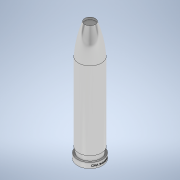
# Autodesk Inventor part: Bala do revólver
Saved by Autodesk Inventor 2021 (Build 250183000, 183)
## iProperties
Created: 2020-11-05
Part Number: Bala do revólver
Material: Liga de Nickel-Copper 400
Document SubType Name: Modeling
Designer: Bruno
Density: 8.83 g/cm^3
Appearance: Cromado - Polido
Author: Bruno
Autodesk Inventor part; units mm, degrees
note: some values were not read from the file. Chosen so that the rebuilt part matches the saved one: direction of "Relevo1".
ref_plane "XY Plane" through (0, 0, 0) normal (0, 0, 1) x (1, 0, 0)
sketch "Esboço1" plane through (0, 0, 0) normal (0, 1, 0) x (-1, 0, 0)
  circle A0 centre (0, 0) radius 3.5
  dimension "d0" = 7
  constraints: 1 centre point, 1 coincident
  measures "d0" diameter of A0
extrude "Extrusão1" add sketch "Esboço1" along normal blind 1.5
sketch "Esboço2" plane through (0, 1.5, 0) normal (0, 1, 0) x (1, 0, 0)
  circle A0 centre (0, 0) radius 3
  dimension "d3" = 6
  constraints: 1 centre point, 1 coincident
  measures "d3" diameter of A0
extrude "Extrusão2" add sketch "Esboço2" along normal blind 1.5
sketch "Esboço3" plane through (0, 3, 0) normal (0, 1, 0) x (1, 0, 0)
  circle A0 centre (0, 0) radius 3.25
  dimension "d6" = 6.5
  constraints: 1 centre point, 1 coincident
  measures "d6" diameter of A0
extrude "Extrusão3" add sketch "Esboço3" along normal blind 22
sketch "Esboço4" plane through (0, 0, 0) normal (0, 0, 1) x (1, 0, 0)
  line L0 (0, 25) -> (0, 36.9625)
  line L1 (0, -7.4277) -> (0, 44.566) projected
  line L2 (3.25, 25) -> (-3.25, 25) projected
  line L3 (0, 25) -> (3.25, 25)
  arc A0 (3.25, 25) -> (0, 36.9625) centre (-25.6934, 23.5594) ccw
  point P0 (0, 0)
  constraints: 4 end point, 2 point on circle, 1 centre point, 1 horizontal, 1 vertical
revolve "Revolução2" add sketch "Esboço4" angle 360 about axis through (0, -10, 0) along (0, 1, 0)
ref_plane "Plano de trabalho1" through (0, 36.963, 0) normal (0, 1, 0) x (-1, 0, 0)
sketch "Esboço5" plane through (0, 36.963, 0) normal (0, 1, 0) x (-1, 0, 0)
  circle A0 centre (0, 0) radius 1.5
  dimension "d12" = 3
  constraints: 1 centre point, 1 coincident
  measures "d12" diameter of A0
extrude "Extrusão4" cut sketch "Esboço5" against normal blind 3.963
sketch "Esboço6" plane through (0, 0, 0) normal (0, -1, 0) x (1, 0, 0)
  circle A0 centre (0, 0) radius 1.25
  dimension "d15" = 2.5
  constraints: 1 centre point, 1 coincident
  measures "d15" diameter of A0
extrude "Extrusão5" cut sketch "Esboço6" against normal blind 0.5
sketch "Esboço7" plane through (0, 0.5, 0) normal (0, -1, 0) x (1, 0, 0)
  circle A0 centre (0, 0) radius 1.25 projected
  circle A1 centre (0, 0) radius 1.2
  dimension "d18" = 2.4
  constraints: 1 centre point, 1 coincident
  measures "d18" diameter of A1
extrude "Extrusão6" add sketch "Esboço7" along normal blind 0.5 contours A1
sketch "Esboço8" plane through (0, 0, 0) normal (0, -1, 0) x (1, 0, 0)
  circle A0 centre (0, 0) radius 0.05
  dimension "d21" = 0.1
  constraints: 1 centre point, 1 coincident
  measures "d21" diameter of A0
extrude "Extrusão7" cut sketch "Esboço8" against normal blind 0.5
ref_plane "Plano de trabalho2" through (3.5, 0, 0) normal (1, 0, 0) x (0, 1, 0)
sketch "Esboço10" plane through (3.5, 0, 0) normal (1, 0, 0) x (0, 1, 0)
  line L0 (0.9718, 2.3396) -> (0.9718, -2.2443) construction
  line L1 (0.9718, -2.2443) -> (0.439, -2.2443) construction
  line L2 (0.439, -2.2443) -> (0.439, 2.3396) construction
  line L3 (0.439, 2.3396) -> (0.9718, 2.3396) construction
  spline S0 degree 2 poles (0.4406, 2.0936) (0.4406, 2.1422) (0.4735, 2.2245) (0.5063, 2.2545) knots 0 0 0 1 2 2 2
  spline S1 degree 2 poles (0.5063, 2.2545) (0.5387, 2.2845) (0.6359, 2.3173) (0.6991, 2.3173) knots 0 0 0 1 2 2 2
  spline S2 degree 2 poles (0.6991, 2.3173) (0.7619, 2.3173) (0.8551, 2.2853) (0.8896, 2.2549) knots 0 0 0 1 2 2 2
  spline S3 degree 2 poles (0.8896, 2.2549) (0.9232, 2.2249) (0.9585, 2.1431) (0.9585, 2.0924) knots 0 0 0 1 2 2 2
  spline S4 degree 2 poles (0.9585, 2.0924) (0.9585, 2.0673) (0.9512, 2.0231) (0.9455, 2.0045) knots 0 0 0 1 2 2 2
  spline S5 degree 2 poles (0.9455, 2.0045) (0.9402, 1.9883) (0.9252, 1.9546) (0.9163, 1.938) knots 0 0 0 1 2 2 2
  line L4 (0.9163, 1.938) -> (0.8361, 1.938)
  line L5 (0.8361, 1.938) -> (0.8361, 1.9433)
  spline S6 degree 2 poles (0.8361, 1.9433) (0.8442, 1.9522) (0.8669, 1.9798) (0.8778, 1.9996) knots 0 0 0 1 2 2 2
  spline S7 degree 2 poles (0.8778, 1.9996) (0.8884, 2.0187) (0.9017, 2.0636) (0.9017, 2.0928) knots 0 0 0 1 2 2 2
  spline S8 degree 2 poles (0.9017, 2.0928) (0.9017, 2.1248) (0.8754, 2.182) (0.8503, 2.2034) knots 0 0 0 1 2 2 2
  spline S9 degree 2 poles (0.8503, 2.2034) (0.8247, 2.2245) (0.7474, 2.248) (0.6991, 2.248) knots 0 0 0 1 2 2 2
  spline S10 degree 2 poles (0.6991, 2.248) (0.6477, 2.248) (0.5735, 2.2233) (0.548, 2.2018) knots 0 0 0 1 2 2 2
  spline S11 degree 2 poles (0.548, 2.2018) (0.5233, 2.1807) (0.4982, 2.1244) (0.4982, 2.0928) knots 0 0 0 1 2 2 2
  spline S12 degree 2 poles (0.4982, 2.0928) (0.4982, 2.064) (0.5124, 2.015) (0.5229, 1.996) knots 0 0 0 1 2 2 2
  spline S13 degree 2 poles (0.5229, 1.996) (0.5334, 1.9777) (0.5553, 1.9506) (0.563, 1.9429) knots 0 0 0 1 2 2 2
  line L6 (0.563, 1.9429) -> (0.563, 1.938)
  line L7 (0.563, 1.938) -> (0.4836, 1.938)
  spline S14 degree 2 poles (0.4836, 1.938) (0.4759, 1.9546) (0.4617, 1.9838) (0.4552, 2.0045) knots 0 0 0 1 2 2 2
  spline S15 degree 2 poles (0.4552, 2.0045) (0.4479, 2.0264) (0.4406, 2.0636) (0.4406, 2.0936) knots 0 0 0 1 2 2 2
  line L8 (0.4495, 1.4473) -> (0.4495, 1.5138)
  line L9 (0.4495, 1.5138) -> (0.8803, 1.5138)
  line L10 (0.8803, 1.5138) -> (0.5873, 1.6443)
  line L11 (0.5873, 1.6443) -> (0.5873, 1.6848)
  line L12 (0.5873, 1.6848) -> (0.8803, 1.814)
  line L13 (0.8803, 1.814) -> (0.4495, 1.814)
  line L14 (0.4495, 1.814) -> (0.4495, 1.876)
  line L15 (0.4495, 1.876) -> (0.9495, 1.876)
  line L16 (0.9495, 1.876) -> (0.9495, 1.7853)
  line L17 (0.9495, 1.7853) -> (0.6712, 1.6605)
  line L18 (0.6712, 1.6605) -> (0.9495, 1.5397)
  line L19 (0.9495, 1.5397) -> (0.9495, 1.4473)
  line L20 (0.9495, 1.4473) -> (0.4495, 1.4473)
  line L21 (0.4495, 1.3999) -> (0.9495, 1.2314)
  line L22 (0.9495, 1.2314) -> (0.9495, 1.1495)
  line L23 (0.9495, 1.1495) -> (0.4495, 0.981)
  line L24 (0.4495, 0.981) -> (0.4495, 1.0511)
  line L25 (0.4495, 1.0511) -> (0.5893, 1.0965)
  line L26 (0.5893, 1.0965) -> (0.5893, 1.2873)
  line L27 (0.5893, 1.2873) -> (0.4495, 1.3327)
  line L28 (0.4495, 1.3327) -> (0.4495, 1.3999)
  line L29 (0.6461, 1.1147) -> (0.8815, 1.1921)
  line L30 (0.8815, 1.1921) -> (0.6461, 1.2691)
  line L31 (0.6461, 1.2691) -> (0.6461, 1.1147)
  line L32 (0.4495, 0.5446) -> (0.4495, 0.7383)
  line L33 (0.4495, 0.7383) -> (0.5006, 0.7383)
  line L34 (0.5006, 0.7383) -> (0.5006, 0.6747)
  line L35 (0.5006, 0.6747) -> (0.8985, 0.6747)
  line L36 (0.8985, 0.6747) -> (0.8985, 0.7383)
  line L37 (0.8985, 0.7383) -> (0.9495, 0.7383)
  line L38 (0.9495, 0.7383) -> (0.9495, 0.5446)
  line L39 (0.9495, 0.5446) -> (0.8985, 0.5446)
  line L40 (0.8985, 0.5446) -> (0.8985, 0.6082)
  line L41 (0.8985, 0.6082) -> (0.5006, 0.6082)
  line L42 (0.5006, 0.6082) -> (0.5006, 0.5446)
  line L43 (0.5006, 0.5446) -> (0.4495, 0.5446)
  line L44 (0.4495, 0.1726) -> (0.4495, 0.2358)
  line L45 (0.4495, 0.2358) -> (0.6635, 0.2358)
  spline S16 degree 2 poles (0.6635, 0.2358) (0.6894, 0.2358) (0.734, 0.2407) (0.7474, 0.248) knots 0 0 0 1 2 2 2
  spline S17 degree 2 poles (0.7474, 0.248) (0.7615, 0.2557) (0.7753, 0.2832) (0.7753, 0.3067) knots 0 0 0 1 2 2 2
  spline S18 degree 2 poles (0.7753, 0.3067) (0.7753, 0.3302) (0.7502, 0.3801) (0.7299, 0.404) knots 0 0 0 1 2 2 2
  line L46 (0.7299, 0.404) -> (0.4495, 0.404)
  line L47 (0.4495, 0.404) -> (0.4495, 0.4672)
  line L48 (0.4495, 0.4672) -> (0.8247, 0.4672)
  line L49 (0.8247, 0.4672) -> (0.8247, 0.404)
  line L50 (0.8247, 0.404) -> (0.783, 0.404)
  spline S19 degree 2 poles (0.783, 0.404) (0.8085, 0.3756) (0.8353, 0.3209) (0.8353, 0.2901) knots 0 0 0 1 2 2 2
  spline S20 degree 2 poles (0.8353, 0.2901) (0.8353, 0.235) (0.7624, 0.1726) (0.6931, 0.1726) knots 0 0 0 1 2 2 2
  line L51 (0.6931, 0.1726) -> (0.4495, 0.1726)
  line L52 (0.4495, -0.2046) -> (0.4495, -0.1414)
  line L53 (0.4495, -0.1414) -> (0.4876, -0.1414)
  spline S21 degree 2 poles (0.4876, -0.1414) (0.4755, -0.1268) (0.4593, -0.1053) (0.4524, -0.0907) knots 0 0 0 1 2 2 2
  spline S22 degree 2 poles (0.4524, -0.0907) (0.4459, -0.0774) (0.439, -0.0486) (0.439, -0.0296) knots 0 0 0 1 2 2 2
  spline S23 degree 2 poles (0.439, -0.0296) (0.439, 0.0012) (0.4645, 0.0531) (0.4893, 0.0713) knots 0 0 0 1 2 2 2
  spline S24 degree 2 poles (0.4893, 0.0713) (0.514, 0.0896) (0.5869, 0.1098) (0.6343, 0.1098) knots 0 0 0 1 2 2 2
  spline S25 degree 2 poles (0.6343, 0.1098) (0.6837, 0.1098) (0.7559, 0.0843) (0.783, 0.062) knots 0 0 0 1 2 2 2
  spline S26 degree 2 poles (0.783, 0.062) (0.8073, 0.0414) (0.8353, -0.0166) (0.8353, -0.0486) knots 0 0 0 1 2 2 2
  spline S27 degree 2 poles (0.8353, -0.0486) (0.8353, -0.0766) (0.8227, -0.1183) (0.8098, -0.1414) knots 0 0 0 1 2 2 2
  line L54 (0.8098, -0.1414) -> (0.9718, -0.1414)
  line L55 (0.9718, -0.1414) -> (0.9718, -0.2046)
  line L56 (0.9718, -0.2046) -> (0.4495, -0.2046)
  line L57 (0.5407, -0.1414) -> (0.7575, -0.1414)
  spline S28 degree 2 poles (0.7575, -0.1414) (0.7688, -0.1179) (0.7773, -0.0806) (0.7773, -0.0591) knots 0 0 0 1 2 2 2
  spline S29 degree 2 poles (0.7773, -0.0591) (0.7773, -0.0105) (0.7044, 0.0446) (0.6355, 0.0446) knots 0 0 0 1 2 2 2
  spline S30 degree 2 poles (0.6355, 0.0446) (0.5691, 0.0446) (0.499, 0.0025) (0.499, -0.0441) knots 0 0 0 1 2 2 2
  spline S31 degree 2 poles (0.499, -0.0441) (0.499, -0.0689) (0.5217, -0.1191) (0.5407, -0.1414) knots 0 0 0 1 2 2 2
  line L58 (0.4495, -0.5879) -> (0.4495, -0.5247)
  line L59 (0.4495, -0.5247) -> (0.4909, -0.5247)
  spline S32 degree 2 poles (0.4909, -0.5247) (0.4653, -0.4955) (0.439, -0.4433) (0.439, -0.4108) knots 0 0 0 1 2 2 2
  spline S33 degree 2 poles (0.439, -0.4108) (0.439, -0.3865) (0.4552, -0.3432) (0.4726, -0.3274) knots 0 0 0 1 2 2 2
  spline S34 degree 2 poles (0.4726, -0.3274) (0.4901, -0.3112) (0.5431, -0.2933) (0.5812, -0.2933) knots 0 0 0 1 2 2 2
  line L60 (0.5812, -0.2933) -> (0.8247, -0.2933)
  line L61 (0.8247, -0.2933) -> (0.8247, -0.3565)
  line L62 (0.8247, -0.3565) -> (0.6108, -0.3565)
  spline S35 degree 2 poles (0.6108, -0.3565) (0.5808, -0.3565) (0.5415, -0.361) (0.5269, -0.3687) knots 0 0 0 1 2 2 2
  spline S36 degree 2 poles (0.5269, -0.3687) (0.5124, -0.3764) (0.499, -0.4027) (0.499, -0.4275) knots 0 0 0 1 2 2 2
  spline S37 degree 2 poles (0.499, -0.4275) (0.499, -0.4505) (0.5253, -0.5028) (0.5444, -0.5247) knots 0 0 0 1 2 2 2
  line L63 (0.5444, -0.5247) -> (0.8247, -0.5247)
  line L64 (0.8247, -0.5247) -> (0.8247, -0.5879)
  line L65 (0.8247, -0.5879) -> (0.4495, -0.5879)
  spline S38 degree 2 poles (0.4406, -0.7808) (0.4406, -0.7431) (0.4609, -0.6779) (0.4722, -0.6564) knots 0 0 0 1 2 2 2
  line L66 (0.4722, -0.6564) -> (0.5431, -0.6564)
  line L67 (0.5431, -0.6564) -> (0.5431, -0.6596)
  spline S39 degree 2 poles (0.5431, -0.6596) (0.5367, -0.6677) (0.5213, -0.6896) (0.5128, -0.7078) knots 0 0 0 1 2 2 2
  spline S40 degree 2 poles (0.5128, -0.7078) (0.5051, -0.7236) (0.4937, -0.7625) (0.4937, -0.7832) knots 0 0 0 1 2 2 2
  spline S41 degree 2 poles (0.4937, -0.7832) (0.4937, -0.7982) (0.5006, -0.8326) (0.5063, -0.8407) knots 0 0 0 1 2 2 2
  spline S42 degree 2 poles (0.5063, -0.8407) (0.514, -0.8525) (0.5314, -0.863) (0.5492, -0.863) knots 0 0 0 1 2 2 2
  spline S43 degree 2 poles (0.5492, -0.863) (0.5715, -0.863) (0.5946, -0.8387) (0.6023, -0.8075) knots 0 0 0 1 2 2 2
  spline S44 degree 2 poles (0.6023, -0.8075) (0.6051, -0.7954) (0.6132, -0.7565) (0.6177, -0.7398) knots 0 0 0 1 2 2 2
  spline S45 degree 2 poles (0.6177, -0.7398) (0.6303, -0.6969) (0.6821, -0.658) (0.719, -0.658) knots 0 0 0 1 2 2 2
  spline S46 degree 2 poles (0.719, -0.658) (0.77, -0.658) (0.8337, -0.7346) (0.8337, -0.7978) knots 0 0 0 1 2 2 2
  spline S47 degree 2 poles (0.8337, -0.7978) (0.8337, -0.829) (0.8183, -0.8922) (0.8065, -0.9137) knots 0 0 0 1 2 2 2
  line L68 (0.8065, -0.9137) -> (0.7388, -0.9137)
  line L69 (0.7388, -0.9137) -> (0.7388, -0.9104)
  spline S48 degree 2 poles (0.7388, -0.9104) (0.7583, -0.8861) (0.7806, -0.827) (0.7806, -0.7966) knots 0 0 0 1 2 2 2
  spline S49 degree 2 poles (0.7806, -0.7966) (0.7806, -0.7654) (0.7542, -0.7224) (0.7279, -0.7224) knots 0 0 0 1 2 2 2
  spline S50 degree 2 poles (0.7279, -0.7224) (0.704, -0.7224) (0.6809, -0.748) (0.6736, -0.7763) knots 0 0 0 1 2 2 2
  spline S51 degree 2 poles (0.6736, -0.7763) (0.67, -0.7901) (0.6627, -0.8249) (0.6582, -0.844) knots 0 0 0 1 2 2 2
  spline S52 degree 2 poles (0.6582, -0.844) (0.6477, -0.8853) (0.5995, -0.9275) (0.5577, -0.9275) knots 0 0 0 1 2 2 2
  spline S53 degree 2 poles (0.5577, -0.9275) (0.5334, -0.9275) (0.4905, -0.9084) (0.4747, -0.8898) knots 0 0 0 1 2 2 2
  spline S54 degree 2 poles (0.4747, -0.8898) (0.4581, -0.8699) (0.4406, -0.8193) (0.4406, -0.7808) knots 0 0 0 1 2 2 2
  spline S55 degree 2 poles (0.4423, -1.0997) (0.4423, -1.0482) (0.501, -0.9903) (0.5646, -0.9903) knots 0 0 0 1 2 2 2
  line L70 (0.5646, -0.9903) -> (0.7725, -0.9903)
  line L71 (0.7725, -0.9903) -> (0.7725, -0.9477)
  line L72 (0.7725, -0.9477) -> (0.8247, -0.9477)
  line L73 (0.8247, -0.9477) -> (0.8247, -0.9903)
  line L74 (0.8247, -0.9903) -> (0.9325, -0.9903)
  line L75 (0.9325, -0.9903) -> (0.9325, -1.0535)
  line L76 (0.9325, -1.0535) -> (0.8247, -1.0535)
  line L77 (0.8247, -1.0535) -> (0.8247, -1.1698)
  line L78 (0.8247, -1.1698) -> (0.7725, -1.1698)
  line L79 (0.7725, -1.1698) -> (0.7725, -1.0535)
  line L80 (0.7725, -1.0535) -> (0.5938, -1.0535)
  spline S56 degree 2 poles (0.5938, -1.0535) (0.5654, -1.0535) (0.5342, -1.0555) (0.5209, -1.0624) knots 0 0 0 1 2 2 2
  spline S57 degree 2 poles (0.5209, -1.0624) (0.5091, -1.068) (0.4974, -1.0936) (0.4974, -1.1155) knots 0 0 0 1 2 2 2
  spline S58 degree 2 poles (0.4974, -1.1155) (0.4974, -1.1309) (0.5067, -1.1596) (0.5095, -1.1661) knots 0 0 0 1 2 2 2
  line L81 (0.5095, -1.1661) -> (0.5095, -1.1698)
  line L82 (0.5095, -1.1698) -> (0.4528, -1.1698)
  spline S59 degree 2 poles (0.4528, -1.1698) (0.4479, -1.1519) (0.4423, -1.1155) (0.4423, -1.0997) knots 0 0 0 1 2 2 2
  line L83 (0.7571, -1.4153) -> (0.7571, -1.4121)
  spline S60 degree 2 poles (0.7571, -1.4121) (0.7591, -1.4048) (0.7599, -1.389) (0.7599, -1.378) knots 0 0 0 1 2 2 2
  spline S61 degree 2 poles (0.7599, -1.378) (0.7599, -1.3525) (0.7376, -1.3022) (0.7158, -1.2796) knots 0 0 0 1 2 2 2
  line L84 (0.7158, -1.2796) -> (0.4495, -1.2796)
  line L85 (0.4495, -1.2796) -> (0.4495, -1.2163)
  line L86 (0.4495, -1.2163) -> (0.8247, -1.2163)
  line L87 (0.8247, -1.2163) -> (0.8247, -1.2796)
  line L88 (0.8247, -1.2796) -> (0.7688, -1.2796)
  spline S62 degree 2 poles (0.7688, -1.2796) (0.7996, -1.314) (0.8247, -1.3655) (0.8247, -1.3898) knots 0 0 0 1 2 2 2
  spline S63 degree 2 poles (0.8247, -1.3898) (0.8247, -1.3995) (0.8239, -1.4092) (0.8227, -1.4153) knots 0 0 0 1 2 2 2
  line L89 (0.8227, -1.4153) -> (0.7571, -1.4153)
  line L90 (0.4495, -1.5287) -> (0.4495, -1.4655)
  line L91 (0.4495, -1.4655) -> (0.8247, -1.4655)
  line L92 (0.8247, -1.4655) -> (0.8247, -1.5287)
  line L93 (0.8247, -1.5287) -> (0.4495, -1.5287)
  line L94 (0.8871, -1.5332) -> (0.8871, -1.4615)
  line L95 (0.8871, -1.4615) -> (0.9528, -1.4615)
  line L96 (0.9528, -1.4615) -> (0.9528, -1.5332)
  line L97 (0.9528, -1.5332) -> (0.8871, -1.5332)
  spline S64 degree 2 poles (0.441, -1.7844) (0.441, -1.6945) (0.5419, -1.5956) (0.6351, -1.5956) knots 0 0 0 1 2 2 2
  spline S65 degree 2 poles (0.6351, -1.5956) (0.7267, -1.5956) (0.8353, -1.6916) (0.8353, -1.769) knots 0 0 0 1 2 2 2
  spline S66 degree 2 poles (0.8353, -1.769) (0.8353, -1.8039) (0.815, -1.8578) (0.7935, -1.8776) knots 0 0 0 1 2 2 2
  spline S67 degree 2 poles (0.7935, -1.8776) (0.7721, -1.8979) (0.7101, -1.9193) (0.6651, -1.9193) knots 0 0 0 1 2 2 2
  line L98 (0.6651, -1.9193) -> (0.6307, -1.9193)
  line L99 (0.6307, -1.9193) -> (0.6307, -1.6596)
  spline S68 degree 2 poles (0.6307, -1.6596) (0.5654, -1.6596) (0.4961, -1.7253) (0.4961, -1.7836) knots 0 0 0 1 2 2 2
  spline S69 degree 2 poles (0.4961, -1.7836) (0.4961, -1.8043) (0.5055, -1.8444) (0.5128, -1.8606) knots 0 0 0 1 2 2 2
  spline S70 degree 2 poles (0.5128, -1.8606) (0.5209, -1.8776) (0.535, -1.9011) (0.5415, -1.9088) knots 0 0 0 1 2 2 2
  line L100 (0.5415, -1.9088) -> (0.5415, -1.9125)
  line L101 (0.5415, -1.9125) -> (0.4726, -1.9125)
  spline S71 degree 2 poles (0.4726, -1.9125) (0.4682, -1.9015) (0.4552, -1.8683) (0.4516, -1.8553) knots 0 0 0 1 2 2 2
  spline S72 degree 2 poles (0.4516, -1.8553) (0.4463, -1.8371) (0.441, -1.8071) (0.441, -1.7844) knots 0 0 0 1 2 2 2
  spline S73 degree 2 poles (0.6789, -1.8578) (0.7044, -1.8569) (0.7417, -1.8464) (0.7542, -1.8363) knots 0 0 0 1 2 2 2
  spline S74 degree 2 poles (0.7542, -1.8363) (0.7684, -1.8253) (0.7834, -1.7909) (0.7834, -1.7654) knots 0 0 0 1 2 2 2
  spline S75 degree 2 poles (0.7834, -1.7654) (0.7834, -1.7403) (0.7684, -1.705) (0.7538, -1.6904) knots 0 0 0 1 2 2 2
  spline S76 degree 2 poles (0.7538, -1.6904) (0.7388, -1.6762) (0.7028, -1.6616) (0.6789, -1.6596) knots 0 0 0 1 2 2 2
  line L102 (0.6789, -1.6596) -> (0.6789, -1.8578)
  spline S77 degree 2 poles (0.4406, -2.0847) (0.4406, -2.047) (0.4609, -1.9817) (0.4722, -1.9603) knots 0 0 0 1 2 2 2
  line L103 (0.4722, -1.9603) -> (0.5431, -1.9603)
  line L104 (0.5431, -1.9603) -> (0.5431, -1.9635)
  spline S78 degree 2 poles (0.5431, -1.9635) (0.5367, -1.9716) (0.5213, -1.9935) (0.5128, -2.0117) knots 0 0 0 1 2 2 2
  spline S79 degree 2 poles (0.5128, -2.0117) (0.5051, -2.0275) (0.4937, -2.0664) (0.4937, -2.0871) knots 0 0 0 1 2 2 2
  spline S80 degree 2 poles (0.4937, -2.0871) (0.4937, -2.1021) (0.5006, -2.1365) (0.5063, -2.1446) knots 0 0 0 1 2 2 2
  spline S81 degree 2 poles (0.5063, -2.1446) (0.514, -2.1564) (0.5314, -2.1669) (0.5492, -2.1669) knots 0 0 0 1 2 2 2
  spline S82 degree 2 poles (0.5492, -2.1669) (0.5715, -2.1669) (0.5946, -2.1426) (0.6023, -2.1114) knots 0 0 0 1 2 2 2
  spline S83 degree 2 poles (0.6023, -2.1114) (0.6051, -2.0992) (0.6132, -2.0604) (0.6177, -2.0437) knots 0 0 0 1 2 2 2
  spline S84 degree 2 poles (0.6177, -2.0437) (0.6303, -2.0008) (0.6821, -1.9619) (0.719, -1.9619) knots 0 0 0 1 2 2 2
  spline S85 degree 2 poles (0.719, -1.9619) (0.77, -1.9619) (0.8337, -2.0385) (0.8337, -2.1017) knots 0 0 0 1 2 2 2
  spline S86 degree 2 poles (0.8337, -2.1017) (0.8337, -2.1329) (0.8183, -2.1961) (0.8065, -2.2176) knots 0 0 0 1 2 2 2
  line L105 (0.8065, -2.2176) -> (0.7388, -2.2176)
  line L106 (0.7388, -2.2176) -> (0.7388, -2.2143)
  spline S87 degree 2 poles (0.7388, -2.2143) (0.7583, -2.19) (0.7806, -2.1309) (0.7806, -2.1005) knots 0 0 0 1 2 2 2
  spline S88 degree 2 poles (0.7806, -2.1005) (0.7806, -2.0693) (0.7542, -2.0263) (0.7279, -2.0263) knots 0 0 0 1 2 2 2
  spline S89 degree 2 poles (0.7279, -2.0263) (0.704, -2.0263) (0.6809, -2.0518) (0.6736, -2.0802) knots 0 0 0 1 2 2 2
  spline S90 degree 2 poles (0.6736, -2.0802) (0.67, -2.094) (0.6627, -2.1288) (0.6582, -2.1479) knots 0 0 0 1 2 2 2
  spline S91 degree 2 poles (0.6582, -2.1479) (0.6477, -2.1892) (0.5995, -2.2313) (0.5577, -2.2313) knots 0 0 0 1 2 2 2
  spline S92 degree 2 poles (0.5577, -2.2313) (0.5334, -2.2313) (0.4905, -2.2123) (0.4747, -2.1937) knots 0 0 0 1 2 2 2
  spline S93 degree 2 poles (0.4747, -2.1937) (0.4581, -2.1738) (0.4406, -2.1232) (0.4406, -2.0847) knots 0 0 0 1 2 2 2
  point P0 (0, 0)
  constraints: 2 other
emboss "Relevo1" sketch "Esboço10" operation cut depth 1 direction (-1, 0, 0)
